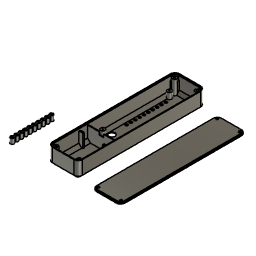
storm (Autodesk Fusion 360 design; units mm, degrees)
Autodesk Fusion 360 part; units mm, degrees
sketch "Sketch1" plane through (0, 0, 0) normal (0, 0, 1) x (1, 0, 0)
  line L0 (-1, -0.8) -> (1, -0.8)
  line L1 (-1, 0.8) -> (1, 0.8)
  circle A0 centre (0, 0) radius 2.5
  arc A1 (-1, 0.8) -> (-1, -0.8) centre (-1, 0) ccw
  arc A2 (1, -0.8) -> (1, 0.8) centre (1, 0) ccw
  arc A3 (1, 5.2) -> (1, 6.8) centre (1, 6) ccw
  line L2 (-1, 5.2) -> (1, 5.2)
  circle A4 centre (0, 6) radius 2.5
  arc A5 (-1, 6.8) -> (-1, 5.2) centre (-1, 6) ccw
  line L3 (-1, 6.8) -> (1, 6.8)
  line L4 (1, 3.7087) -> (1, 2.2913)
  line L5 (-1, 2.2913) -> (-1, 3.7087)
  line L6 (-1, 11.2) -> (1, 11.2)
  line L7 (-1, 12.8) -> (1, 12.8)
  arc A6 (-1, 12.8) -> (-1, 11.2) centre (-1, 12) ccw
  arc A7 (1, 11.2) -> (1, 12.8) centre (1, 12) ccw
  line L8 (-1, 8.2913) -> (-1, 9.7087)
  circle A8 centre (0, 12) radius 2.5
  line L9 (1, 9.7087) -> (1, 8.2913)
  line L10 (1, 21.7087) -> (1, 20.2913)
  line L11 (1, 15.7087) -> (1, 14.2913)
  line L12 (-1, 24.8) -> (1, 24.8)
  circle A9 centre (0, 18) radius 2.5
  line L13 (-1, 14.2913) -> (-1, 15.7087)
  line L14 (-1, 20.2913) -> (-1, 21.7087)
  circle A10 centre (0, 24) radius 2.5
  arc A11 (-1, 18.8) -> (-1, 17.2) centre (-1, 18) ccw
  line L15 (-1, 17.2) -> (1, 17.2)
  arc A12 (1, 17.2) -> (1, 18.8) centre (1, 18) ccw
  line L16 (-1, 18.8) -> (1, 18.8)
  arc A13 (1, 23.2) -> (1, 24.8) centre (1, 24) ccw
  arc A14 (-1, 24.8) -> (-1, 23.2) centre (-1, 24) ccw
  line L17 (-1, 23.2) -> (1, 23.2)
  line L18 (-1, 26.2913) -> (-1, 27.7087)
  circle A15 centre (0, 30) radius 2.5
  line L19 (1, 27.7087) -> (1, 26.2913)
  line L20 (-1, 30.8) -> (1, 30.8)
  arc A16 (-1, 30.8) -> (-1, 29.2) centre (-1, 30) ccw
  arc A17 (1, 29.2) -> (1, 30.8) centre (1, 30) ccw
  line L21 (-1, 36.8) -> (1, 36.8)
  arc A18 (-1, 36.8) -> (-1, 35.2) centre (-1, 36) ccw
  circle A19 centre (0, 36) radius 2.5
  arc A20 (1, 35.2) -> (1, 36.8) centre (1, 36) ccw
  line L22 (-1, 35.2) -> (1, 35.2)
  line L23 (1, 33.7087) -> (1, 32.2913)
  line L24 (-1, 29.2) -> (1, 29.2)
  line L25 (-1, 32.2913) -> (-1, 33.7087)
  arc A21 (1, 47.2) -> (1, 48.8) centre (1, 48) ccw
  line L26 (1, 39.7087) -> (1, 38.2913)
  line L27 (-1, 47.2) -> (1, 47.2)
  arc A22 (-1, 54.8) -> (-1, 53.2) centre (-1, 54) ccw
  line L28 (-1, 44.2913) -> (-1, 45.7087)
  line L29 (-1, 53.2) -> (1, 53.2)
  line L30 (-1, 42.8) -> (1, 42.8)
  line L31 (1, 51.7087) -> (1, 50.2913)
  circle A23 centre (0, 54) radius 2.5
  arc A24 (1, 53.2) -> (1, 54.8) centre (1, 54) ccw
  arc A25 (-1, 42.8) -> (-1, 41.2) centre (-1, 42) ccw
  arc A26 (-1, 48.8) -> (-1, 47.2) centre (-1, 48) ccw
  line L32 (1, 45.7087) -> (1, 44.2913)
  circle A27 centre (0, 42) radius 2.5
  line L33 (-1, 50.2913) -> (-1, 51.7087)
  arc A28 (1, 41.2) -> (1, 42.8) centre (1, 42) ccw
  circle A29 centre (0, 48) radius 2.5
  line L34 (-1, 38.2913) -> (-1, 39.7087)
  line L35 (-1, 41.2) -> (1, 41.2)
  line L36 (-1, 48.8) -> (1, 48.8)
  line L37 (-1, 54.8) -> (1, 54.8)
  dimension "d1" = 0.8
  dimension "d2" = 0.8
  dimension "d3" = 5
  dimension "d4" = 5
  dimension "d5" = 5
  dimension "d6" = 5
  dimension "d7" = 5
  dimension "d8" = 5
  dimension "d9" = 5
  dimension "d10" = 5
  dimension "d11" = 5
  dimension "d12" = 5
  constraint horizontal L0
  constraint coincident A0.centre origin
  constraint horizontal L2
  constraint vertical L4
  constraint vertical L5
  constraint coincident A4 L4.start
  constraint coincident A4 L5.end
  constraint coincident A0 L5.start
  constraint coincident A0 L4.end
  constraint horizontal L6
  constraint vertical L9
  constraint vertical L8
  constraint coincident L9.start A8
  constraint coincident L8.end A8
  constraint horizontal L15
  constraint vertical L11
  constraint vertical L13
  constraint coincident L11.start A9
  constraint coincident L13.end A9
  constraint horizontal L17
  constraint vertical L10
  constraint vertical L14
  constraint coincident L10.start A10
  constraint coincident L14.end A10
  constraint horizontal L24
  constraint vertical L19
  constraint vertical L18
  constraint coincident L19.start A15
  constraint coincident L18.end A15
  constraint horizontal L22
  constraint vertical L23
  constraint vertical L25
  constraint coincident L23.start A19
  constraint coincident L25.end A19
  constraint horizontal L35
  constraint vertical L26
  constraint vertical L34
  constraint coincident L26.start A27
  constraint coincident L34.end A27
  constraint horizontal L27
  constraint vertical L32
  constraint vertical L28
  constraint coincident L32.start A29
  constraint coincident L28.end A29
  constraint horizontal L29
  constraint vertical L31
  constraint vertical L33
  constraint coincident L31.start A23
  constraint coincident L33.end A23
  measures "d1" distance of A0.centre L0
  measures "d2" distance of A0.centre L1
  measures "d3" diameter of A0
  measures "d4" diameter of A4
  measures "d5" diameter of A8
  measures "d6" diameter of A9
  measures "d7" diameter of A10
  measures "d8" diameter of A15
  measures "d9" diameter of A19
  measures "d10" diameter of A27
  measures "d11" diameter of A29
  measures "d12" diameter of A23
extrude "Extrude1" add sketch "Sketch1" along normal blind 7 makes body 1
sketch "Sketch2" plane through (0, 0, 0) normal (0, 0, 1) x (1, 0, 0)
  line L0 (55.2, 0) -> (84.8, 0)
  line L1 (90.6, 5.8) -> (90.6, 168.4)
  line L2 (84.8, 174.2) -> (55.2, 174.2)
  line L3 (49.4, 168.4) -> (49.4, 5.8)
  line L4 (56, 1.6) -> (84, 1.6)
  line L5 (89, 6.6) -> (89, 167.6)
  line L6 (84, 172.6) -> (56, 172.6)
  line L7 (51, 167.6) -> (51, 6.6)
  line L8 (55.5, 0.6) -> (84.5, 0.6)
  line L9 (90, 6.1) -> (90, 168.1)
  line L10 (84.5, 173.6) -> (55.5, 173.6)
  line L11 (50, 168.1) -> (50, 6.1)
  line L12 (51, 52.6) -> (89, 52.6)
  line L13 (51, 53.6) -> (89, 53.6)
  circle A0 centre (84.5, 160.6) radius 3
  circle A1 centre (55.5, 160.6) radius 3
  circle A2 centre (55.5, 69.1) radius 3
  circle A3 centre (84.5, 69.1) radius 3
  line L14 (67, 53.6) -> (67, 52.6)
  line L15 (73, 53.6) -> (73, 52.6)
  circle A4 centre (54.5, 5.6) radius 3
  circle A5 centre (85.5, 5.6) radius 3
  line L16 (56.5, 7.8361) -> (56.5, 3.3639)
  line L17 (83.5, 7.8361) -> (83.5, 3.3639)
  circle A6 centre (54.5, 5.6) radius 1
  circle A7 centre (85.5, 5.6) radius 1
  circle A8 centre (58, 153.1) radius 1.85
  circle A9 centre (58, 147.1) radius 1.85
  circle A10 centre (58, 141.1) radius 1.85
  circle A11 centre (58, 135.1) radius 1.85
  circle A12 centre (58, 129.1) radius 1.85
  circle A13 centre (58, 123.1) radius 1.85
  circle A14 centre (58, 117.1) radius 1.85
  circle A15 centre (58, 111.1) radius 1.85
  circle A16 centre (58, 105.1) radius 1.85
  circle A17 centre (58, 99.1) radius 1.85
  circle A18 centre (82, 153.1) radius 1.85
  circle A19 centre (82, 147.1) radius 1.85
  circle A20 centre (82, 141.1) radius 1.85
  circle A21 centre (82, 135.1) radius 1.85
  circle A22 centre (82, 129.1) radius 1.85
  circle A23 centre (82, 123.1) radius 1.85
  circle A24 centre (82, 117.1) radius 1.85
  circle A25 centre (82, 111.1) radius 1.85
  circle A26 centre (82, 105.1) radius 1.85
  circle A27 centre (82, 99.1) radius 1.85
  circle A28 centre (80.5, 61.1) radius 3.75
  circle A29 centre (80.5, 77.6) radius 4.25
  circle A30 centre (59.5, 77.6) radius 4.25
  circle A31 centre (59, 61.1) radius 4.25
  circle A32 centre (54.5, 168.6) radius 3
  circle A33 centre (85.5, 168.6) radius 3
  line L18 (89, 42.6) -> (83.5, 42.6)
  line L19 (83.5, 42.6) -> (83.5, 40.6)
  line L20 (83.5, 40.6) -> (89, 40.6)
  line L21 (89, 40.6) -> (89, 42.6)
  line L22 (51, 42.6) -> (56.5, 42.6)
  line L23 (56.5, 42.6) -> (56.5, 40.6)
  line L24 (56.5, 40.6) -> (51, 40.6)
  line L25 (51, 40.6) -> (51, 42.6)
  arc A34 (56, 172.6) -> (51, 167.6) centre (56, 167.6) ccw
  arc A35 (55.5, 173.6) -> (50, 168.1) centre (55.5, 168.1) ccw
  arc A36 (55.2, 174.2) -> (49.4, 168.4) centre (55.2, 168.4) ccw
  arc A37 (89, 167.6) -> (84, 172.6) centre (84, 167.6) ccw
  arc A38 (90, 168.1) -> (84.5, 173.6) centre (84.5, 168.1) ccw
  arc A39 (90.6, 168.4) -> (84.8, 174.2) centre (84.8, 168.4) ccw
  arc A40 (84, 1.6) -> (89, 6.6) centre (84, 6.6) ccw
  arc A41 (84.5, 0.6) -> (90, 6.1) centre (84.5, 6.1) ccw
  arc A42 (84.8, 0) -> (90.6, 5.8) centre (84.8, 5.8) ccw
  arc A43 (51, 6.6) -> (56, 1.6) centre (56, 6.6) ccw
  arc A44 (50, 6.1) -> (55.5, 0.6) centre (55.5, 6.1) ccw
  arc A45 (49.4, 5.8) -> (55.2, 0) centre (55.2, 5.8) ccw
  line L26 (56.9857, 172.6) -> (55, 172.6)
  line L27 (51, 168.6) -> (51, 166)
  line L28 (51, 166) -> (56.9857, 166)
  line L29 (56.9857, 166) -> (56.9857, 172.6)
  arc A46 (55, 172.6) -> (51, 168.6) centre (55, 168.6) ccw
  line L30 (82.9977, 172.6) -> (85, 172.6)
  line L31 (89, 168.6) -> (89, 166)
  line L32 (89, 166) -> (82.9977, 166)
  line L33 (82.9977, 166) -> (82.9977, 172.6)
  arc A47 (89, 168.6) -> (85, 172.6) centre (85, 168.6) ccw
  line L34 (83.5, 1.6) -> (85, 1.6)
  line L35 (89, 5.6) -> (89, 7.5)
  line L36 (89, 7.5) -> (83.5, 7.5)
  line L37 (83.5, 7.5) -> (83.5, 1.6)
  arc A48 (85, 1.6) -> (89, 5.6) centre (85, 5.6) ccw
  line L38 (56.5, 1.6) -> (55, 1.6)
  line L39 (51, 5.6) -> (51, 7.5)
  line L40 (51, 7.5) -> (56.5, 7.5)
  line L41 (56.5, 7.5) -> (56.5, 1.6)
  arc A49 (51, 5.6) -> (55, 1.6) centre (55, 5.6) ccw
  point P0 (49.4, 0)
  point P1 (90.6, 0)
  point P2 (49.4, 174.2)
  dimension "d15" = 41.2
  dimension "d16" = 174.2
  dimension "d17" = 1.6
  dimension "d18" = 1.6
  dimension "d19" = 1.6
  dimension "d20" = 1.6
  dimension "d21" = 0.6
  dimension "d22" = 0.6
  dimension "d23" = 0.6
  dimension "d24" = 0.6
  dimension "d25" = 51
  dimension "d26" = 1
  dimension "d27" = 6
  dimension "d28" = 12
  dimension "d29" = 4.5
  dimension "d30" = 6
  dimension "d31" = 12
  dimension "d32" = 4.5
  dimension "d33" = 6
  dimension "d34" = 6
  dimension "d35" = 91.5
  dimension "d36" = 91.5
  dimension "d37" = 4.5
  dimension "d38" = 4.5
  dimension "d39" = 16
  dimension "d40" = 16
  dimension "d41" = 6
  dimension "d42" = 6
  dimension "d43" = 3.5
  dimension "d44" = 3.5
  dimension "d45" = 4
  dimension "d46" = 4
  dimension "d47" = 27
  dimension "d49" = 7.1
  dimension "d50" = 2
  dimension "d51" = 2
  dimension "d52" = 3.7
  dimension "d53" = 19.5
  dimension "d54" = 7
  dimension "d55" = 3.7
  dimension "d56" = 6
  dimension "d57" = 3.7
  dimension "d58" = 6
  dimension "d59" = 3.7
  dimension "d60" = 6
  dimension "d61" = 3.7
  dimension "d62" = 6
  dimension "d63" = 3.7
  dimension "d64" = 6
  dimension "d65" = 3.7
  dimension "d66" = 6
  dimension "d67" = 3.7
  dimension "d68" = 3.7
  dimension "d69" = 3.7
  dimension "d70" = 6
  dimension "d71" = 6
  dimension "d72" = 6
  dimension "d73" = 3.7
  dimension "d74" = 7
  dimension "d75" = 19.5
  dimension "d76" = 3.7
  dimension "d77" = 3.7
  dimension "d78" = 3.7
  dimension "d79" = 3.7
  dimension "d80" = 3.7
  dimension "d81" = 3.7
  dimension "d82" = 3.7
  dimension "d83" = 3.7
  dimension "d84" = 3.7
  dimension "d85" = 6
  dimension "d86" = 6
  dimension "d87" = 6
  dimension "d88" = 6
  dimension "d89" = 6
  dimension "d90" = 6
  dimension "d91" = 6
  dimension "d92" = 6
  dimension "d93" = 6
  dimension "d94" = 7.5
  dimension "d95" = 8.5
  dimension "d96" = 8.5
  dimension "d97" = 8.5
  dimension "d98" = 7.5
  dimension "d99" = 7.5
  dimension "d100" = 8
  dimension "d101" = 8.5
  dimension "d102" = 8.5
  dimension "d103" = 8.5
  dimension "d104" = 24
  dimension "d105" = 24
  dimension "d106" = 6
  dimension "d107" = 6
  dimension "d108" = 3.5
  dimension "d109" = 3.5
  dimension "d110" = 4
  dimension "d111" = 4
  dimension "d140" = 5.5
  dimension "d141" = 2
  dimension "d142" = 10
  dimension "d143" = 2
  dimension "d144" = 5.5
  dimension "d145" = 10
  dimension "d182" = 5
  dimension "d183" = 5.5
  dimension "d184" = 5.8
  dimension "d185" = 5
  dimension "d186" = 5.5
  dimension "d187" = 5.8
  dimension "d188" = 5
  dimension "d189" = 5.5
  dimension "d190" = 5.8
  dimension "d191" = 5
  dimension "d192" = 5.5
  dimension "d193" = 5.8
  dimension "d223" = 4
  dimension "d224" = 4
  dimension "d225" = 4
  dimension "d226" = 4
  constraint horizontal L0
  constraint vertical L1
  constraint horizontal L2
  constraint vertical L3
  constraint perpendicular L3 L4
  constraint perpendicular L0 L5
  constraint perpendicular L5 L6
  constraint perpendicular L4 L7
  constraint perpendicular L5 L8
  constraint perpendicular L6 L9
  constraint perpendicular L3 L10
  constraint perpendicular L8 L11
  constraint coincident L7 L12.start
  constraint coincident L5 L12.end
  constraint perpendicular L5 L12
  constraint coincident L7 L13.start
  constraint coincident L5 L13.end
  constraint perpendicular L5 L13
  constraint coincident L13 L14.start
  constraint coincident L12 L14.end
  constraint perpendicular L12 L14
  constraint coincident L13 L15.start
  constraint coincident L12 L15.end
  constraint perpendicular L12 L15
  constraint coincident A4 L16.start
  constraint coincident A4 L16.end
  constraint parallel L7 L16
  constraint coincident A5 L17.start
  constraint coincident A5 L17.end
  constraint parallel L16 L17
  constraint concentric A4 A6
  constraint concentric A5 A7
  constraint horizontal L18
  constraint vertical L19
  constraint horizontal L20
  constraint vertical L21
  constraint coincident L5 L18.start
  constraint horizontal L22
  constraint vertical L23
  constraint horizontal L24
  constraint vertical L25
  constraint coincident L7 L22.start
  constraint tangent L7 A34
  constraint tangent L6 A34
  constraint tangent L10 A35
  constraint tangent L11 A35
  constraint coincident P2 L2
  constraint coincident P2 L3
  constraint tangent L2 A36
  constraint tangent L3 A36
  constraint tangent L6 A37
  constraint tangent L5 A37
  constraint tangent L10 A38
  constraint tangent L9 A38
  constraint tangent L2 A39
  constraint tangent L1 A39
  constraint tangent L5 A40
  constraint tangent L4 A40
  constraint tangent L9 A41
  constraint tangent L8 A41
  constraint coincident P1 L1
  constraint coincident P1 L0
  constraint tangent L1 A42
  constraint tangent L0 A42
  constraint tangent L7 A43
  constraint tangent L4 A43
  constraint tangent L11 A44
  constraint tangent L8 A44
  constraint coincident P0 L3
  constraint coincident P0 L0
  constraint tangent L3 A45
  constraint tangent L0 A45
  constraint horizontal L26
  constraint vertical L27
  constraint horizontal L28
  constraint vertical L29
  constraint coincident L7 L27.end
  constraint coincident L6 L26.start
  constraint tangent L26 A46
  constraint tangent L27 A46
  constraint horizontal L30
  constraint vertical L31
  constraint horizontal L32
  constraint vertical L33
  constraint coincident L5 L31.end
  constraint coincident L6 L30.start
  constraint tangent L30 A47
  constraint tangent L31 A47
  constraint horizontal L34
  constraint vertical L35
  constraint horizontal L36
  constraint vertical L37
  constraint coincident L5 L35.end
  constraint coincident L4 L34.start
  constraint tangent L34 A48
  constraint tangent L35 A48
  constraint horizontal L38
  constraint vertical L39
  constraint horizontal L40
  constraint vertical L41
  constraint coincident L7 L39.end
  constraint coincident L4 L38.start
  constraint tangent L38 A49
  constraint tangent L39 A49
  measures "d15" distance of P0 P1
  measures "d16" distance of P0 P2
  measures "d17" distance of L1 L5
  measures "d18" distance of L3 L7
  measures "d19" distance of L0 L4
  measures "d20" distance of L2 L6
  measures "d21" distance of L1 L9
  measures "d22" distance of L3 L11
  measures "d23" distance of L2 L10
  measures "d24" distance of L0 L8
  measures "d25" distance of L4 L12
  measures "d26" distance of L12 L13
  measures "d27" diameter of A0
  measures "d28" distance of L6 A0.centre
  measures "d29" distance of L5 A0.centre
  measures "d30" diameter of A1
  measures "d31" distance of L6 A1.centre
  measures "d32" distance of L7 A1.centre
  measures "d33" diameter of A2
  measures "d34" diameter of A3
  measures "d35" vertical distance of A0.centre A3.centre
  measures "d36" vertical distance of A1.centre A2.centre
  measures "d37" distance of L5 A3.centre
  measures "d38" distance of L7 A2.centre
  measures "d39" distance of L7 L14
  measures "d40" distance of L5 L15
  measures "d41" diameter of A4
  measures "d42" diameter of A5
  measures "d43" distance of L7 A4.centre
  measures "d44" distance of L5 A5.centre
  measures "d45" distance of L4 A5.centre
  measures "d46" distance of L4 A4.centre
  measures "d47" distance of L16 L17
  measures "d49" distance of L1 L17
  measures "d50" diameter of A6
  measures "d51" diameter of A7
  measures "d52" diameter of A8
  measures "d53" distance of L6 A8.centre
  measures "d54" distance of L7 A8.centre
  measures "d55" diameter of A9
  measures "d56" distance of A8.centre A9.centre
  measures "d57" diameter of A10
  measures "d58" distance of A9.centre A10.centre
  measures "d59" diameter of A11
  measures "d60" distance of A10.centre A11.centre
  measures "d61" diameter of A12
  measures "d62" distance of A11.centre A12.centre
  measures "d63" diameter of A13
  measures "d64" distance of A12.centre A13.centre
  measures "d65" diameter of A14
  measures "d66" distance of A13.centre A14.centre
  measures "d67" diameter of A15
  measures "d68" diameter of A16
  measures "d69" diameter of A17
  measures "d70" distance of A14.centre A15.centre
  measures "d71" distance of A15.centre A16.centre
  measures "d72" distance of A16.centre A17.centre
  measures "d73" diameter of A18
  measures "d74" distance of L5 A18.centre
  measures "d75" distance of L6 A18.centre
  measures "d76" diameter of A19
  measures "d77" diameter of A20
  measures "d78" diameter of A21
  measures "d79" diameter of A22
  measures "d80" diameter of A23
  measures "d81" diameter of A24
  measures "d82" diameter of A25
  measures "d83" diameter of A26
  measures "d84" diameter of A27
  measures "d85" distance of A18.centre A19.centre
  measures "d86" distance of A19.centre A20.centre
  measures "d87" distance of A20.centre A21.centre
  measures "d88" distance of A21.centre A22.centre
  measures "d89" distance of A22.centre A23.centre
  measures "d90" distance of A23.centre A24.centre
  measures "d91" distance of A24.centre A25.centre
  measures "d92" distance of A25.centre A26.centre
  measures "d93" distance of A26.centre A27.centre
  measures "d94" diameter of A28
  measures "d95" diameter of A29
  measures "d96" diameter of A30
  measures "d97" diameter of A31
  measures "d98" distance of L13 A28.centre
  measures "d99" distance of L13 A31.centre
  measures "d100" distance of L7 A31.centre
  measures "d101" distance of L5 A28.centre
  measures "d102" distance of L5 A29.centre
  measures "d103" distance of L7 A30.centre
  measures "d104" distance of L13 A29.centre
  measures "d105" distance of L13 A30.centre
  measures "d106" diameter of A32
  measures "d107" diameter of A33
  measures "d108" distance of L7 A32.centre
  measures "d109" distance of L5 A33.centre
  measures "d110" distance of L6 A33.centre
  measures "d111" distance of L6 A32.centre
  measures "d140" distance of L5 L19
  measures "d141" distance of L18 L20
  measures "d142" distance of L12 L18
  measures "d143" distance of L22 L24
  measures "d144" distance of L7 L23
  measures "d145" distance of L12 L22
  measures "d182" radius of A34
  measures "d183" radius of A35
  measures "d184" radius of A36
  measures "d185" radius of A37
  measures "d186" radius of A38
  measures "d187" radius of A39
  measures "d188" radius of A40
  measures "d189" radius of A41
  measures "d190" radius of A42
  measures "d191" radius of A43
  measures "d192" radius of A44
  measures "d193" radius of A45
  measures "d223" radius of A46
  measures "d224" radius of A47
  measures "d225" radius of A48
  measures "d226" radius of A49
extrude "Extrude2" add sketch "Sketch2" along normal blind 21.5 separate body contours L0 L1 L2 L3 A36 A39 A42 A45 makes body 2
extrude "Extrude3" add sketch "Sketch2" along normal blind 20.5 contours A43 L38 L39 A49 | A40 L34 L35 A48 | A34 L26 L27 A46 | A37 L30 L31 A47 | L8 L9 L10 L11 A35 A38 A41 A44 bodies 2
extrude "Extrude4" add sketch "Sketch2" along normal blind 20.5 contours L7 L12 L13 L14 | L5 L12 L13 L15 bodies 2
extrude "Extrude5" add sketch "Sketch2" along normal blind 1 contours L4 L7 A4 A43 L38 L39 L40 L41 | L4 L5 L7 L12 A4 A5 L18 L19 L20 L22 L23 L24 L36 L37 L40 L41 | L4 L5 A5 A40 L34 L35 L36 L37 | L7 L22 L23 L24 L25 | L5 L18 L19 L20 L21 | L5 L6 L7 L13 A32 A33 L28 L29 L32 L33 | L6 L7 A32 A34 L26 L27 L28 L29 | A32 L28 L29 | L5 L6 A33 A37 L30 L31 L32 L33 | A33 L32 L33 picked at (56.7696, 166.3511) picked at (83.2164, 166.3602) bodies 2
extrude "Extrude6" add sketch "Sketch2" along normal blind 16.5 contours L12 L13 L14 L15 bodies 2
extrude "Extrude7" add sketch "Sketch2" along normal blind 15.5 contours A4 L16 L40 L41 | A5 L17 L36 L37 | A4 L16 L40 | A5 L17 L36 | A32 L28 | A32 L28 L29 | A32 L29 | A33 L32 L33 | A33 L32 | A33 L33 | A6 | A7 picked at (55.0067, 168.4782) picked at (84.9083, 168.8541) bodies 2
extrude "Extrude8" add sketch "Sketch2" along normal blind 9.5 contours A0 | A1 | A2 | A3 bodies 2
sketch "Sketch3" plane through (0, 0, 9.5) normal (0, 0, 1) x (-1, 0, 0)
  circle A0 centre (-55.5, -160.6) radius 3
  circle A1 centre (-55.5, -160.6) radius 0.9
  circle A2 centre (-84.5, -160.5) radius 0.9
  circle A3 centre (-55.5, -69) radius 0.9
  circle A4 centre (-84.5, -69) radius 0.9
  dimension "d126" = 1.8
  dimension "d127" = 1.8
  dimension "d128" = 1.8
  dimension "d129" = 1.8
  constraint concentric A0 A1
  measures "d126" diameter of A1
  measures "d127" diameter of A2
  measures "d128" diameter of A3
  measures "d129" diameter of A4
extrude "Extrude9" cut sketch "Sketch3" against normal blind 6 contours A1 | A2 | A3 | A4 bodies 2
sketch "Sketch4" plane through (0, 0, 15.5) normal (0, 0, 1) x (-1, 0, 0)
  circle A0 centre (-54.5, -168.6) radius 3
  circle A1 centre (-54.5, -5.6) radius 1.25
  circle A2 centre (-85.5, -5.6) radius 1.25
  circle A3 centre (-85.5, -168.6) radius 1.25
  circle A4 centre (-54.5, -168.6) radius 1.25
  dimension "d132" = 2.5
  dimension "d133" = 2.5
  dimension "d134" = 2.5
  dimension "d135" = 2.5
  constraint concentric A0 A4
  measures "d132" diameter of A1
  measures "d133" diameter of A2
  measures "d134" diameter of A3
  measures "d135" diameter of A4
extrude "Extrude10" cut sketch "Sketch4" against normal blind 10 contours A1 | A2 | A3 | A4 bodies 2
extrude "Extrude11" add sketch "Sketch2" along normal blind 1 contours A4 L16 L41 | A5 L17 L37 bodies 2
extrude "Extrude12" add 4 faces at (83.75, 5.6, 15.5) (56.25, 5.6, 15.5) (87.5715, 169.8319, 15.5) (52.1574, 169.1666, 15.5) along direction (0, 0, 1) blind 5 on bodies 2 bodies 2
extrude "Extrude13" add sketch "Sketch2" along normal blind 19.5 contours L7 L22 L23 L24 L25 | L5 L18 L19 L20 L21 bodies 2
sketch "Sketch5" plane through (0, 0, 0) normal (0, 0, 1) x (1, 0, 0)
  line L0 (116, 0) -> (143, 0)
  line L1 (149, 6) -> (149, 166)
  line L2 (143, 172) -> (116, 172)
  line L3 (110, 166) -> (110, 6)
  line L4 (116.6, 1) -> (142.4, 1)
  line L5 (148, 6.6) -> (148, 165.4)
  line L6 (142.4, 171) -> (116.6, 171)
  line L7 (111, 165.4) -> (111, 6.6)
  circle A0 centre (145, 167.5) radius 1.4
  circle A1 centre (114, 167.5) radius 1.4
  circle A2 centre (145, 4.5) radius 1.4
  circle A3 centre (114, 4.5) radius 1.4
  arc A4 (148, 165.4) -> (142.4, 171) centre (142.4, 165.4) ccw
  arc A5 (149, 166) -> (143, 172) centre (143, 166) ccw
  arc A6 (116.6, 171) -> (111, 165.4) centre (116.6, 165.4) ccw
  arc A7 (116, 172) -> (110, 166) centre (116, 166) ccw
  arc A8 (142.4, 1) -> (148, 6.6) centre (142.4, 6.6) ccw
  arc A9 (143, 0) -> (149, 6) centre (143, 6) ccw
  arc A10 (111, 6.6) -> (116.6, 1) centre (116.6, 6.6) ccw
  arc A11 (110, 6) -> (116, 0) centre (116, 6) ccw
  point P0 (110, 0)
  point P1 (149, 0)
  point P2 (110, 172)
  dimension "d150" = 39
  dimension "d151" = 172
  dimension "d152" = 1
  dimension "d153" = 1
  dimension "d154" = 1
  dimension "d155" = 1
  dimension "d156" = 2.8
  dimension "d157" = 2.8
  dimension "d158" = 2.8
  dimension "d159" = 2.8
  dimension "d160" = 3.5
  dimension "d161" = 3
  dimension "d162" = 3
  dimension "d163" = 3.5
  dimension "d164" = 3.5
  dimension "d165" = 3
  dimension "d166" = 3
  dimension "d167" = 3.5
  dimension "d208" = 5.6
  dimension "d209" = 6
  dimension "d210" = 5.6
  dimension "d211" = 6
  dimension "d212" = 5.6
  dimension "d213" = 6
  dimension "d214" = 5.6
  dimension "d215" = 6
  constraint horizontal L0
  constraint vertical L1
  constraint horizontal L2
  constraint vertical L3
  constraint perpendicular L3 L4
  constraint perpendicular L2 L5
  constraint perpendicular L1 L6
  constraint perpendicular L4 L7
  constraint tangent L5 A4
  constraint tangent L6 A4
  constraint tangent L2 A5
  constraint tangent L1 A5
  constraint tangent L6 A6
  constraint tangent L7 A6
  constraint coincident P2 L2
  constraint coincident P2 L3
  constraint tangent L2 A7
  constraint tangent L3 A7
  constraint tangent L5 A8
  constraint tangent L4 A8
  constraint coincident P1 L1
  constraint coincident P1 L0
  constraint tangent L1 A9
  constraint tangent L0 A9
  constraint tangent L7 A10
  constraint tangent L4 A10
  constraint coincident P0 L3
  constraint coincident P0 L0
  constraint tangent L3 A11
  constraint tangent L0 A11
  measures "d150" distance of P0 P1
  measures "d151" distance of P0 P2
  measures "d152" distance of L1 L5
  measures "d153" distance of L3 L7
  measures "d154" distance of L0 L4
  measures "d155" distance of L2 L6
  measures "d156" diameter of A0
  measures "d157" diameter of A1
  measures "d158" diameter of A2
  measures "d159" diameter of A3
  measures "d160" distance of L4 A3.centre
  measures "d161" distance of L7 A3.centre
  measures "d162" distance of L5 A2.centre
  measures "d163" distance of L4 A2.centre
  measures "d164" distance of L6 A0.centre
  measures "d165" distance of L5 A0.centre
  measures "d166" distance of L7 A1.centre
  measures "d167" distance of L6 A1.centre
  measures "d208" radius of A4
  measures "d209" radius of A5
  measures "d210" radius of A6
  measures "d211" radius of A7
  measures "d212" radius of A8
  measures "d213" radius of A9
  measures "d214" radius of A10
  measures "d215" radius of A11
extrude "Extrude24" add sketch "Sketch5" along normal blind 1.2 separate body contours L0 L1 L2 L3 A5 A7 A9 A11 | L4 L5 L6 L7 A4 A6 A8 A10 makes body 3
chamfer "Chamfer4" distance 1 angle 45 1 edges at (143.6947, 168.0063, 0) on bodies 3
chamfer "Chamfer5" distance 1 angle 45 3 edges at (112.6947, 168.0063, 0) (143.6947, 5.0063, 0) (112.6947, 5.0063, 0) on bodies 3
extrude "Extrude25" add sketch "Sketch5" along normal blind 2.2 contours L4 L5 L6 L7 A4 A6 A8 A10 bodies 3
chamfer "Chamfer6" distance 2 angle 45 4 edges at (143.6947, 168.0063, 0) (112.6947, 168.0063, 0) (112.6947, 5.0063, 0) (143.6947, 5.0063, 0) on bodies 3
extrude "Extrude26" add sketch "Sketch2" along normal blind 17 contours L4 L7 A4 A43 L38 L39 L40 L41 | A43 L38 L39 A49 | L4 L5 A5 A40 L34 L35 L36 L37 | A40 L34 L35 A48 | L6 L7 A32 A34 L26 L27 L28 L29 | A34 L26 L27 A46 | L5 L6 A33 A37 L30 L31 L32 L33 | A37 L30 L31 A47 bodies 2
chamfer "Chamfer7" distance 4 angle 45 8 edges at (51, 109.8, 1) (69.9917, 172.6, 1) (89, 109.8, 1) (89, 47.6, 1) (89, 24.05, 1) (51, 24.05, 1) (51, 47.6, 1) (70, 1.6, 1) on bodies 2
chamfer "Chamfer8" distance 4 angle 45 8 edges at (49.4, 87.1, 0) (51.0988, 1.6988, 0) (70, 0, 0) (88.9012, 1.6988, 0) (90.6, 87.1, 0) (88.9012, 172.5012, 0) (70, 174.2, 0) (51.0988, 172.5012, 0) on bodies 2
extrude "Extrude27" add 1 faces at (49.6, 60.1, 21.5) along direction (0, 0, 1) blind 1.5 on bodies 2 bodies 2
extrude "Extrude28" add 1 faces at (89.6667, 75.9333, 20.5) along direction (0, 0, 1) blind 1.5 on bodies 2 bodies 2
sketch "Sketch7" plane through (0, 0, 22) normal (0, 0, 1) x (-1, 0, 0)
  arc A0 (-51, -6.6) -> (-56, -1.6) centre (-56, -6.6) ccw
  line L0 (-51, -6.6) -> (-51, -52.6)
  line L1 (-51, -52.6) -> (-67, -52.6)
  line L2 (-67, -52.6) -> (-67, -53.6)
  line L3 (-67, -53.6) -> (-51, -53.6)
  line L4 (-51, -53.6) -> (-51, -167.6)
  arc A1 (-56, -172.6) -> (-51, -167.6) centre (-56, -167.6) ccw
  line L5 (-56, -172.6) -> (-84, -172.6)
  arc A2 (-89, -167.6) -> (-84, -172.6) centre (-84, -167.6) ccw
  line L6 (-89, -167.6) -> (-89, -53.6)
  line L7 (-89, -53.6) -> (-73, -53.6)
  line L8 (-73, -53.6) -> (-73, -52.6)
  line L9 (-73, -52.6) -> (-89, -52.6)
  line L10 (-89, -52.6) -> (-89, -6.6)
  arc A3 (-84, -1.6) -> (-89, -6.6) centre (-84, -6.6) ccw
  line L11 (-84, -1.6) -> (-56, -1.6)
  arc A4 (-50, -6.1) -> (-55.5, -0.6) centre (-55.5, -6.1) ccw
  line L12 (-55.5, -0.6) -> (-84.5, -0.6)
  arc A5 (-84.5, -0.6) -> (-90, -6.1) centre (-84.5, -6.1) ccw
  line L13 (-90, -6.1) -> (-90, -168.1)
  arc A6 (-90, -168.1) -> (-84.5, -173.6) centre (-84.5, -168.1) ccw
  line L14 (-84.5, -173.6) -> (-55.5, -173.6)
  arc A7 (-55.5, -173.6) -> (-50, -168.1) centre (-55.5, -168.1) ccw
  line L15 (-50, -168.1) -> (-50, -6.1)
  line L16 (-51, -53.6) -> (-89, -53.6)
  line L17 (-89, -53.6) -> (-89, -52.6)
  line L18 (-89, -52.6) -> (-51, -52.6)
  line L19 (-51, -52.6) -> (-51, -53.6)
  constraint horizontal L16
  constraint vertical L17
  constraint horizontal L18
  constraint vertical L19
  constraint coincident L9.end L10.start
  constraint coincident L3.end L4.start
extrude "Extrude29" cut sketch "Sketch7" against normal blind 1.5 contours L1 L2 L3 L16 L18 L19 | L7 L8 L9 L16 L17 L18 bodies 2
extrude "Extrude14" [suppressed]
extrude "Extrude15" [suppressed]
chamfer "Chamfer1" [suppressed]
extrude "Extrude16" [suppressed]
extrude "Extrude17" [suppressed]
extrude "Extrude18" [suppressed]
extrude "Extrude19" [suppressed]
sketch "Sketch6" plane through (0, 0, 1) normal (0, 0, 1) x (-1, 0, 0)
  circle A0 centre (-80.5, -61.1) radius 3.75
  circle A1 centre (-55.5, -160.6) radius 3
  circle A2 centre (-58, -129.1) radius 1.85
  circle A3 centre (-58, -105.1) radius 1.85
  circle A4 centre (-58, -111.1) radius 1.85
  circle A5 centre (-58, -141.1) radius 1.85
  circle A6 centre (-58, -153.1) radius 1.85
  circle A7 centre (-54.5, -168.6) radius 3
  circle A8 centre (-58, -135.1) radius 1.85
  circle A9 centre (-58, -123.1) radius 1.85
  circle A10 centre (-59.5, -77.6) radius 4.25
  circle A11 centre (-82, -147.1) radius 1.85
  circle A12 centre (-82, -141.1) radius 1.85
  circle A13 centre (-82, -123.1) radius 1.85
  circle A14 centre (-82, -135.1) radius 1.85
  circle A15 centre (-84.5, -69.1) radius 3
  circle A16 centre (-85.5, -168.6) radius 3
  circle A17 centre (-58, -117.1) radius 1.85
  circle A18 centre (-80.5, -77.6) radius 4.25
  circle A19 centre (-84.5, -160.6) radius 3
  circle A20 centre (-82, -153.1) radius 1.85
  circle A21 centre (-82, -105.1) radius 1.85
  circle A22 centre (-82, -129.1) radius 1.85
  circle A23 centre (-58, -99.1) radius 1.85
  circle A24 centre (-82, -117.1) radius 1.85
  circle A25 centre (-58, -147.1) radius 1.85
  circle A26 centre (-55.5, -69.1) radius 3
  circle A27 centre (-82, -99.1) radius 1.85
  circle A28 centre (-59, -61.1) radius 4.25
  circle A29 centre (-82, -111.1) radius 1.85
  arc A30 (-89, -167.6) -> (-84, -172.6) centre (-84, -167.6) ccw
  line L0 (-84, -172.6) -> (-56, -172.6)
  arc A31 (-56, -172.6) -> (-51, -167.6) centre (-56, -167.6) ccw
  line L1 (-51, -167.6) -> (-51, -53.6)
  line L2 (-51, -53.6) -> (-89, -53.6)
  line L3 (-89, -53.6) -> (-89, -167.6)
  line L4 (-51, -166) -> (-57.1175, -166)
  line L5 (-57.1175, -166) -> (-57.1175, -172.6)
  line L6 (-57.1175, -172.6) -> (-55, -172.6)
  line L7 (-51, -168.6) -> (-51, -166)
  arc A32 (-55, -172.6) -> (-51, -168.6) centre (-55, -168.6) ccw
  line L8 (-89, -166) -> (-82.9758, -166)
  line L9 (-82.9758, -166) -> (-82.9758, -172.6)
  line L10 (-82.9758, -172.6) -> (-85, -172.6)
  line L11 (-89, -168.6) -> (-89, -166)
  arc A33 (-89, -168.6) -> (-85, -172.6) centre (-85, -168.6) ccw
  line L12 (-51, -8.5) -> (-56.5, -8.5)
  line L13 (-56.5, -8.5) -> (-56.5, -1.6)
  line L14 (-56.5, -1.6) -> (-55, -1.6)
  line L15 (-51, -5.6) -> (-51, -8.5)
  arc A34 (-51, -5.6) -> (-55, -1.6) centre (-55, -5.6) ccw
  line L16 (-89, -8.5) -> (-83.5, -8.5)
  line L17 (-83.5, -8.5) -> (-83.5, -1.6)
  line L18 (-83.5, -1.6) -> (-85, -1.6)
  line L19 (-89, -5.6) -> (-89, -8.5)
  arc A35 (-85, -1.6) -> (-89, -5.6) centre (-85, -5.6) ccw
  dimension "d194" = 4
  dimension "d195" = 4
  dimension "d196" = 4
  dimension "d197" = 4
  constraint horizontal L4
  constraint vertical L5
  constraint horizontal L6
  constraint vertical L7
  constraint coincident L0 L5.end
  constraint coincident L1 L4.start
  constraint tangent L6 A32
  constraint tangent L7 A32
  constraint horizontal L8
  constraint vertical L9
  constraint horizontal L10
  constraint vertical L11
  constraint coincident L0 L9.end
  constraint coincident L3 L8.start
  constraint tangent L10 A33
  constraint tangent L11 A33
  constraint horizontal L12
  constraint vertical L13
  constraint horizontal L14
  constraint vertical L15
  constraint tangent L15 A34
  constraint tangent L14 A34
  constraint horizontal L16
  constraint vertical L17
  constraint horizontal L18
  constraint vertical L19
  constraint tangent L19 A35
  constraint tangent L18 A35
  measures "d194" radius of A32
  measures "d195" radius of A33
  measures "d196" radius of A34
  measures "d197" radius of A35
extrude "Extrude20" [suppressed]
extrude "Extrude21" [suppressed]
extrude "Extrude22" [suppressed]
chamfer "Chamfer2" [suppressed]
chamfer "Chamfer3" [suppressed]
extrude "Extrude23" [suppressed]
